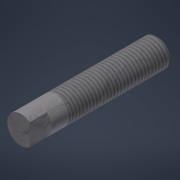
# Autodesk Inventor part: Tornillo de elevación
Saved by Autodesk Inventor 2022 (Build 260153000, 153)
## iProperties
Created: 2021-09-10
Part Number: Tornillo de elevación
Material: Steel, Mild, Welded
Document SubType Name: Modeling
Designer: Andres
Density: 7.85 g/cm^3
Appearance: Weld - Steel Mild
Author: Andres
Autodesk Inventor part; units mm, degrees
ref_plane "YZ Plane" through (0, 0, 0) normal (1, 0, 0) x (0, 1, 0)
ref_plane "XZ Plane" through (0, 0, 0) normal (0, 1, 0) x (-1, 0, 0)
ref_plane "XY Plane" through (0, 0, 0) normal (0, 0, 1) x (1, 0, 0)
sketch "Sketch1" plane through (0, 0, 0) normal (0, 0, 1) x (1, 0, 0)
  circle A0 centre (0, 0) radius 8
  dimension "d0" = 16
  constraints: 1 centre point, 1 coincident
  measures "d0" diameter of A0
extrude "Extrusion1" add sketch "Sketch1" along normal blind 70
thread "Thread1" size "TR16x2" class "7e" standard "ISO Metric Trapezoidal Threads" length 60
sketch "Sketch2" plane through (0, 0, 70) normal (0, 0, 1) x (1, 0, 0)
  circle A0 centre (0, 0) radius 8 projected
  circle A1 centre (0, 0) radius 8 projected
  line L0 (5, 6.245) -> (5, -6.245)
  point P0 (5, -6.245)
  dimension "d7" = 5
  constraints: 2 end point, 2 point on circle, 1 vertical
  measures "d7" distance from line of point (0, 0) L0
extrude "Extrusion2" add sketch "Sketch2" along normal blind 10 contours L0 A0 picked at (-0.3822, -0.6586)
chamfer "Chamfer1" distance 2 angle 45 1 edges at (-8, 0, 0)
body "Solid1"
